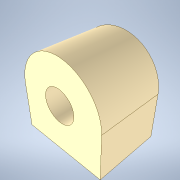
# Autodesk Inventor part: Фиксатор трубки
Saved by Autodesk Inventor 2021.1 (Build 251245010, 245A)
## iProperties
Created: 2026-04-16
Part Number: Фиксатор трубки
Material: Типовые
Document SubType Name: Modeling
Designer: Андрей Тарасов
Density: 1 g/cm^3
Appearance: По умолчанию
Author: Андрей Тарасов
Autodesk Inventor part; units mm, degrees
ref_plane "YZ Plane" through (0, 0, 0) normal (1, 0, 0) x (0, 1, 0)
ref_plane "XZ Plane" through (0, 0, 0) normal (0, 1, 0) x (-1, 0, 0)
ref_plane "XY Plane" through (0, 0, 0) normal (0, 0, 1) x (1, 0, 0)
sketch "Эскиз1" plane through (0, 0, 0) normal (0, 0, 1) x (1, 0, 0)
  circle A0 centre (0, 0) radius 3
  circle A1 centre (0, 0) radius 8
  line L0 (-8, 0) -> (8, 0) construction
  line L1 (8, 0) -> (8, -8.5)
  line L2 (8, -8.5) -> (-8, -8.5)
  line L3 (-8, -8.5) -> (-8, 0)
  line L4 (-8, -2.5) -> (8, -2.5) construction
  dimension "d1" = 16
  dimension "d0" = 6
  dimension "d3" = 6
  dimension "d4" = 2.5
  constraints: 10 end point, 2 coincident, 2 parallel, 2 perpendicular, 2 point on line, 2 vertical, 1 centre point, 1 horizontal, 3 other
  measures "d0" diameter of A0
  measures "d3" distance between parallel lines of L2 L4
  measures "d4" distance from line of point (0, 0) L4
extrude "Выдавливание1" add sketch "Эскиз1" along normal blind 12
